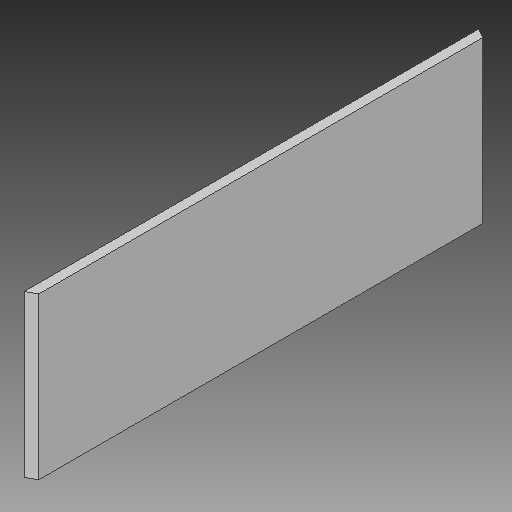
# Autodesk Inventor part: Back Wall
Saved by Autodesk Inventor 2017 (Build 210142000, 142)
## iProperties
Created: 2017-06-10
Part Number: Back Wall
Material: Generic
Document SubType Name: Modeling
Designer: Matthew
Density: 1 g/cm^3
Appearance: Default
Author: Matthew
Autodesk Inventor part; units mm, degrees
ref_plane "YZ Plane" through (0, 0, 0) normal (1, 0, 0) x (0, 1, 0)
ref_plane "XZ Plane" through (0, 0, 0) normal (0, 1, 0) x (-1, 0, 0)
sketch "Sketch1" plane through (0, 0, 0) normal (0, 1, 0) x (-1, 0, 0)
  line L0 (0, 0) -> (3.175, 0)
  line L1 (3.175, 0) -> (3.175, -152.4)
  line L2 (3.175, -152.4) -> (0, -152.4)
  line L3 (0, -152.4) -> (0, 0)
  dimension "d0" = 3.175
  dimension "d1" = 152.4
  constraints: 8 end point, 2 parallel, 1 horizontal, 1 perpendicular
  measures "d0" distance of L1.end L2.end
  measures "d1" distance of L0.end L1.end
extrude "Extrusion1" add sketch "Sketch1" along normal blind 53.975
sketch "Sketch2" plane through (0, 53.975, 0) normal (0, 1, 0) x (1, 0, 0)
  line L0 (-3.175, 152.4) -> (-3.175, 0) projected
  line L1 (-3.175, 0) -> (78.8226, -52.7127)
  line L2 (78.8226, -52.7127) -> (78.8226, -16.7976)
  line L3 (-3.175, 0) -> (11.7687, 8.1586)
  line L4 (0, 0) -> (0, 152.4) projected
  line L5 (0, 1.7334) -> (0, 0)
  line L6 (0, 0) -> (-3.175, 0)
  dimension "d4" = 57.265
  dimension "d5" = 61.368
  constraints: 10 end point, 2 point on line, 1 collinear, 1 parallel, 1 perpendicular
  measures "d4" angle of L2 L1
  measures "d5" angle of L0 L3
ref_plane "Work Plane1" through (0, 0, -76.2) normal (0, 0, -1) x (-1, 0, 0)
extrude "Extrusion2" cut sketch "Sketch2" against normal blind 53.975
mirror "Mirror1" about plane through (0, 0, -76.2) normal (0, 0, -1) of "Extrusion2"
sketch "Sketch3" plane through (-3.175, 0, 0) normal (-1, 0, 0) x (0, 0, 1)
  line L0 (-152.4, 53.975) -> (0, 53.975) projected
  line L1 (-152.4, 0) -> (-152.4, 53.975) projected
  point P0 (0, 0)
  point P1 (-120.65, 44.45)
  point P2 (-31.75, 44.45)
  dimension "d8" = 9.525
  dimension "d9" = 31.75
  dimension "d10" = 31.75
  constraints: 1 horizontal alignment
  measures "d8" distance from line of L0 point (-31.75, 44.45)
  measures "d9" horizontal distance of L0.end point (-31.75, 44.45)
  measures "d10" distance from line of L1 point (-120.65, 44.45)
body "Solid1"
